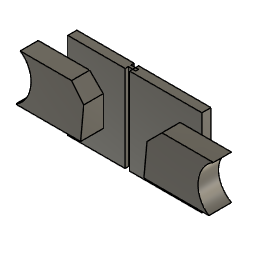
PSP GO R2 v2 (Autodesk Fusion 360 design; units mm, degrees)
Autodesk Fusion 360 part; units mm, degrees
sketch "Boceto1" plane through (0, 0, 0) normal (0, 1, 0) x (1, 0, 0)
  line L0 (3.15, 1.65) -> (-3.15, 1.65)
  line L1 (-3.15, 1.65) -> (-3.15, -1.65)
  line L2 (-3.15, -1.65) -> (3.15, -1.65)
  line L3 (3.15, -1.65) -> (3.15, 1.65)
  arc A0 (-3.15, 1.65) -> (-3.15, -1.65) centre (-3.15, 0) ccw
  arc A1 (3.15, -1.65) -> (3.15, 1.65) centre (3.15, 0) ccw
  line L4 (8.25, 1.45) -> (8.25, 1.65)
  line L5 (-10.9, -2.725) -> (9.9, -2.725)
  line L6 (9.9, -2.725) -> (9.9, 3.025)
  line L7 (9.9, 3.025) -> (-10.9, 3.025)
  line L8 (-10.9, 3.025) -> (-10.9, -2.725)
  line L9 (-8.25, 1.45) -> (8.25, 1.45)
  line L10 (8.25, 1.65) -> (8.25, 1.45)
  line L11 (-8.25, 1.45) -> (-8.25, -1.45)
  line L12 (-8.25, -1.45) -> (8.25, -1.45)
  line L13 (8.25, 1.45) -> (8.25, -1.45)
  line L14 (-5.9, -2.725) -> (-5.9, 3.025)
  line L15 (5.9, -2.725) -> (5.9, 3.025)
  dimension "d5" = 6.3
  dimension "d6" = 3.15
  dimension "d7" = 3.3
  dimension "d77" = 1.65
  dimension "d78" = 16.5
  dimension "d79" = 8.25
  dimension "d80" = 20.8
  dimension "d81" = 10.9
  dimension "d83" = 5.75
  dimension "d84" = 3.025
  dimension "d95" = 2.9
  dimension "d96" = 1.45
  dimension "d102" = 5
  dimension "d103" = 4
  constraint horizontal L0
  constraint perpendicular L0 L1
  constraint perpendicular L1 L2
  constraint perpendicular L0 L3
  constraint tangent L0 A0
  constraint tangent L0 A1
  constraint perpendicular L2 L4
  constraint coincident L4 L10.start
  constraint horizontal L5
  constraint vertical L6
  constraint horizontal L7
  constraint vertical L8
  constraint coincident L9 L4.start
  constraint perpendicular L9 L10
  constraint perpendicular L11 L12
  constraint coincident L12 L13.end
  constraint perpendicular L12 L13
  constraint coincident L5 L14.start
  constraint coincident L7 L14.end
  constraint perpendicular L7 L14
  constraint coincident L5 L15.start
  constraint coincident L7 L15.end
  constraint perpendicular L7 L15
  measures "d5" distance of L1.end L2.end
  measures "d6" horizontal distance of origin L1.end
  measures "d7" distance of L0.end L1.end
  measures "d77" vertical distance of origin L1.end
  measures "d78" distance of L4.start L9.start
  measures "d79" horizontal distance of origin L9.start
  measures "d80" distance of L5.start L5.end
  measures "d81" horizontal distance of origin L7.end
  measures "d83" distance of L5.start L7.end
  measures "d84" vertical distance of origin L7.end
  measures "d95" distance of L9.start L11.end
  measures "d96" vertical distance of origin L11.end
  measures "d102" distance of L7.end L14.end
  measures "d103" distance of L6.end L15.end
extrude "Extruir25" add sketch "Boceto1" along normal blind 0.6 contours L5 L6 L7 L9 L12 L13 L15 | L9 L12 L13 L15 | L9 L11 L12 L14 | L5 L7 L8 L9 L11 L12 L14 makes body 1 at (7.2333, 0, -1.1083) makes body 2 at (-7.5667, 0, 0.8083)
extrude "Extruir23" add sketch "Boceto1" against normal blind 1.5 contours A1 L9 L12 L15 | A0 L9 L12 L14 | L9 L12 L13 L15 | L9 L11 L12 L14 bodies 2 1
sketch "Boceto18" plane through (8.25, 0, 0) normal (1, 0, 0) x (0, 1, 0)
  line L0 (0, 1.45) -> (-1.5, 1.45)
  line L1 (-1.5, 1.45) -> (-1.5, -1.45)
  line L2 (-1.5, -1.45) -> (0, -1.45)
  line L3 (-1.2, 1.45) -> (-1.5, -1.45)
  line L4 (0, -1.45) -> (0, 1.45)
  point P0 (-1.2, 1.45)
  dimension "d98" = 0.3
  constraint coincident L0 P0
  constraint coincident P0 L3.start
  constraint coincident L1.end L2.start
  measures "d98" distance of L0.end P0
extrude "Extruir24" cut sketch "Boceto18" against normal blind 20 contours L0 L1 L3 bodies 2 1
chamfer "Chaflán8" distance 0.9 angle 45 2 edges at (-8.25, -0.6, 1.45) (8.25, -0.6, 1.45) on bodies 1 2
extrude "Extruir27" cut 1 faces at (9.9, 0.2, 0.8083) along direction (-1, 0, 0) blind 0.2 on bodies 1 bodies 1
sketch "Boceto20" plane through (9.7, 0, 0) normal (1, 0, 0) x (0, 1, 0)
  line L0 (0, 2.725) -> (0, -3.025)
  line L1 (0, -3.025) -> (0.6, -3.025)
  line L2 (0.6, -3.025) -> (0.6, 2.725)
  line L3 (0.6, 2.725) -> (0, 2.725)
  line L4 (0.21, 2.725) -> (0.21, -3.025)
  line L5 (0.39, -3.025) -> (0.39, 2.725)
  dimension "d113" = 0.18
  dimension "d114" = 0.6
  dimension "d115" = 0.21
  constraint coincident L3 L4.start
  constraint coincident L1 L4.end
  constraint perpendicular L1 L4
  constraint coincident L1 L5.start
  constraint coincident L3 L5.end
  constraint perpendicular L3 L5
  measures "d113" distance of L4.start L5.end
  measures "d114" distance of L0.start L2.end
  measures "d115" distance of L0.start L4.start
extrude "Extruir26" add sketch "Boceto20" along normal blind 0.5 contours L1 L3 L4 L5 bodies 1
extrude "Extruir28" cut 1 faces at (-10.9, 0.2, -1.1083) along direction (1, 0, 0) blind 0.2 on bodies 2 bodies 2 1
move_body "Desplazar1" bodies 1 to x (1, 0, 0) y (0, 1, 0) z (0, 0, 1) at (-20.7, 0, 0)
equation "d5 = 9.3 mm - 3 mm"
equation "d6 = d5 / 2"
equation "d77 = d7 / 2"
equation "d79 = d78 / 2"
equation "d81 = ( d80 / 2 ) + 0.5 mm"
equation "d84 = ( d83 / 2 ) + 0.15 mm"
equation "d96 = d95 / 2"
equation "d115 = ( d114 - d113 ) / 2"
